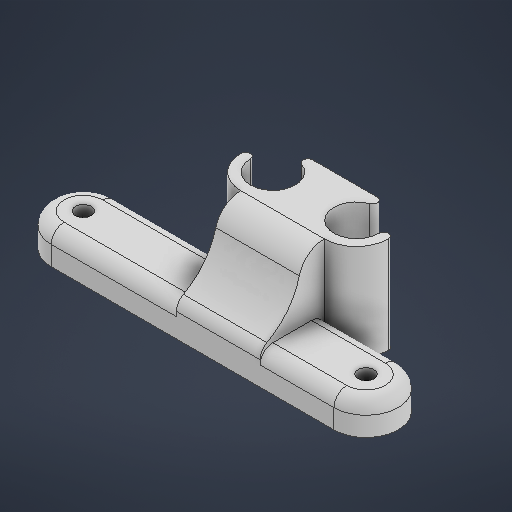
# Autodesk Inventor part: 카메라 하단
Saved by Autodesk Inventor 2026.2 (Build 302298000, 298)
## iProperties
Created: 2026-01-04
Part Number: 카메라 하단
Material: 일반
Document SubType Name: Modeling
Designer: PC
Density: 1 g/cm^3
Appearance: 기본값
Author: PC
Autodesk Inventor part; units mm, degrees
ref_plane "XZ Plane" through (0, 0, 0) normal (0, 1, 0) x (-1, 0, 0)
ref_plane "XY Plane" through (0, 0, 0) normal (0, 0, 1) x (1, 0, 0)
sketch "스케치1" plane through (0, 0, 0) normal (0, 1, 0) x (-1, 0, 0)
  line L0 (0, -14) -> (0, 14) projected
  line L1 (75.6, 0) -> (-75.6, 0) projected
  circle A0 centre (44, 0) radius 1.5
  circle A1 centre (44, 0) radius 10
  line L2 (44, -10) -> (0, -10)
  line L3 (44, 10) -> (0, 10)
  circle A2 centre (-44, 0) radius 1.5
  circle A3 centre (-44, 0) radius 10
  line L4 (-44, -10) -> (0, -10)
  line L5 (-44, 10) -> (0, 10)
  point P0 (0, 0)
  dimension "d0" = 3
  dimension "d1" = 20
  dimension "d2" = 44
  constraints: 8 end point, 4 centre point, 4 point on circle, 4 symmetric about line, 3 point on line, 2 coincident, 2 perpendicular, 2 tangent, 2 other
  measures "d0" diameter of A0
  measures "d1" diameter of A1
  measures "d2" distance of point (0, 0) A0.centre
extrude "돌출1" add sketch "스케치1" along normal blind 10 contours L4 A3 L1 L0 | L0 L1 A1 L2 | L1 A3 L5 L0 | L0 L3 A1 L1 | A1 L1 A0 | A3 L1 A2 | A1 L1 A0 | L1 A2 A3
sketch "스케치2" plane through (0, 10, 0) normal (0, 1, 0) x (1, 0, 0)
  circle A0 centre (-44, 0) radius 1.5 projected
  circle A1 centre (44, 0) radius 1.5 projected
  circle A2 centre (-44, 0) radius 2.5
  circle A3 centre (44, 0) radius 2.5
  point P0 (0, 0)
  dimension "d5" = 5
  dimension "d6" = 5
  constraints: 2 centre point, 2 coincident
  measures "d5" diameter of A2
  measures "d6" diameter of A3
extrude "돌출2" cut sketch "스케치2" against normal blind 5 contours A0 | A1 | A2 | A3
sketch "스케치3" plane through (0, 0, 0) normal (0, -1, 0) x (1, 0, 0)
  line L0 (8, -34.5901) -> (8, 10)
  circle A0 centre (44, 0) radius 1.5 projected
  line L1 (-44, 10) -> (44, 10) projected
  circle A1 centre (21, -20) radius 7
  line L2 (44, -10) -> (-44, -10) projected
  circle A2 centre (21, -20) radius 10
  line L3 (21, -20) -> (11, -20)
  line L4 (21, -20) -> (17.5798, -29.3969)
  line L5 (21, -20) -> (31, -20) construction
  circle A3 centre (18.0928, -27.9874) radius 1.5
  circle A4 centre (29.5, -20) radius 1.5
  line L6 (18.0928, -29.4874) -> (8, -29.4874)
  circle A5 centre (-5, -20) radius 7
  circle A6 centre (-5, -20) radius 10
  circle A7 centre (-2.0928, -27.9874) radius 1.5
  circle A8 centre (-13.5, -20) radius 1.5
  line L7 (-2.0928, -29.4874) -> (8, -29.4874)
  point P0 (0, 0)
  point P1 (18.6059, -26.5778)
  point P2 (28, -20)
  point P3 (21, -10)
  point P4 (-5, -10)
  point P5 (-15, -20)
  point P6 (-12, -20)
  point P7 (-2.6059, -26.5778)
  point P8 (-1.5798, -29.3969)
  point P9 (-1.8394, -29.4874)
  point P10 (17.8394, -29.4874)
  dimension "d9" = 36
  dimension "d10" = 14
  dimension "d11" = 10
  dimension "d12" = 13
  dimension "d13" = 110
  constraints: 12 end point, 6 centre point, 5 symmetric about line, 4 point on line, 3 horizontal, 3 tangent, 2 coincident, 2 point on circle, 2 vertical, 1 equal length, 1 perpendicular, 11 other
  measures "d9" distance from line of L0 A0.centre
  measures "d10" diameter of A1
  measures "d11" distance from line of L2 A1.centre
  measures "d12" distance from line of L0 A1.centre
  measures "d13" angle of L4 L5
extrude "돌출3" add sketch "스케치3" against normal blind 30 contours L7 A6 L2 L0 | L0 L2 A2 L6 | A2 A4 A1 L3 | A6 A7 A5 A8 | A3 L4 | L4 A3 | A2 L3 A1 A3 | A4 | A8 | A7
ref_plane "작업 평면1" through (21, 10, -10) normal (1, 0, 0) x (0, 1, 0)
sketch "스케치4" plane through (21, 10, -10) normal (1, 0, 0) x (0, 1, 0)
  line L0 (20, -10) -> (20, 0) projected
  arc A0 (20, 0) -> (13.903, 7.7704) centre (12, 0) ccw
  arc A1 (0, 20) -> (13.903, 7.7704) centre (18.6605, 27.1963) ccw
  line L1 (20, -3) -> (20, -16.5778) projected
  line L2 (0, 0) -> (20, 0) projected
  line L3 (0, 12.5) -> (0, 7.5) projected
  line L4 (0, 12.5) -> (0, 7.5) projected
  line L5 (0, 20) -> (0, 0) projected
  line L6 (0, 0) -> (0, 20) projected
  point P0 (-10, 10)
  dimension "d16" = 8
  dimension "d17" = 20
  constraints: 4 point on circle, 2 centre point, 2 tangent
  measures "d16" radius of A0
  measures "d17" radius of A1
extrude "돌출4" add sketch "스케치4" against normal blind 26
fillet "모깎기1" radius 4 1 edges at (-24.5, 10, 10)
fillet_without_effect "모깎기2"
